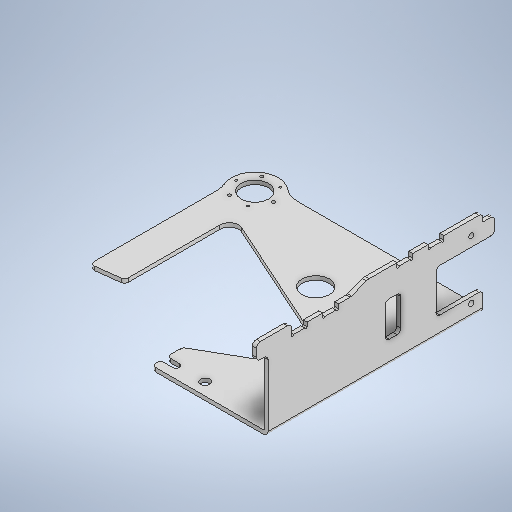
# Autodesk Inventor part: 21-30-220-A
Saved by Autodesk Inventor 2025.2 (Build 292293000, 293)
## iProperties
Created: 2024-11-14
Part Number: 21-30-220-A
Material: Generic
Document SubType Name: Sheet Metal
Designer: Zvonko.Gabric
Density: 1 g/cm^3
Appearance: Default
Sheet Metal Rule: Default
Author: Zvonko.Gabric
Autodesk Inventor part; units mm, degrees
ref_plane "YZ Plane" through (0, 0, 0) normal (1, 0, 0) x (0, 1, 0)
ref_plane "XZ Plane" through (0, 0, 0) normal (0, 1, 0) x (-1, 0, 0)
ref_plane "XY Plane" through (0, 0, 0) normal (0, 0, 1) x (1, 0, 0)
sketch "Sketch1" plane through (0, 0, 0) normal (0, 1, 0) x (-1, 0, 0)
  line L0 (0, 0) -> (140, 0)
  line L1 (145, -5) -> (145, -6)
  line L2 (140, -11) -> (129, -11)
  line L3 (129, -19.6) -> (140, -19.6)
  line L4 (145, -24.6) -> (145, -36.4)
  line L5 (142.4871, -40.7375) -> (88.5077, -71.6894)
  line L6 (257, -199.3068) -> (257, -81.9957)
  line L7 (261.3907, -77.0329) -> (291.3907, -73.3494)
  line L8 (297, -78.3121) -> (297, -235.0208)
  line L9 (0, 0) -> (-79.25, 0)
  line L10 (-84.25, 5) -> (-84.25, 10)
  line L11 (-89.25, 15) -> (-99.25, 15)
  line L12 (-104.25, 10) -> (-104.25, -24.9)
  line L13 (-99.25, -29.9) -> (-90.75, -29.9)
  arc A0 (-84.25, 5) -> (-79.25, 0) centre (-79.25, 5) ccw
  arc A1 (-84.25, 10) -> (-89.25, 15) centre (-89.25, 10) ccw
  arc A2 (-99.25, 15) -> (-104.25, 10) centre (-99.25, 10) ccw
  arc A3 (-104.25, -24.9) -> (-99.25, -29.9) centre (-99.25, -24.9) ccw
  line L14 (-90.75, -32.9) -> (-90.75, -47.1)
  arc A4 (-90.75, -50.1) -> (-90.75, -47.1) centre (-90.75, -48.6) ccw
  line L15 (-90.75, -50.1) -> (-95.85, -50.1)
  line L16 (-95.85, -69.9) -> (-90.75, -69.9)
  arc A5 (-90.75, -72.9) -> (-90.75, -69.9) centre (-90.75, -71.4) ccw
  line L17 (-90.75, -72.9) -> (-90.75, -87.1)
  arc A6 (-90.75, -90.1) -> (-90.75, -87.1) centre (-90.75, -88.6) ccw
  line L18 (-90.75, -90.1) -> (-95.85, -90.1)
  line L19 (-95.85, -90.1) -> (-95.85, -105)
  line L20 (-96.1873, -106.8055) -> (-103.5753, -125.885)
  arc A7 (-96.1873, -106.8055) -> (-95.85, -105) centre (-100.85, -105) ccw
  arc A8 (-103.5753, -125.885) -> (-104.25, -129.496) centre (-94.25, -129.496) ccw
  line L21 (-104.25, -164.9) -> (-99.15, -164.9)
  arc A9 (-99.15, -167.9) -> (-99.15, -164.9) centre (-99.15, -166.4) ccw
  line L22 (-99.15, -167.9) -> (-99.15, -182.1)
  arc A10 (-99.15, -185.1) -> (-99.15, -182.1) centre (-99.15, -183.6) ccw
  line L23 (-99.15, -185.1) -> (-104.25, -185.1)
  line L24 (-104.25, -185.1) -> (-104.25, -204.9)
  line L25 (-104.25, -204.9) -> (-99.15, -204.9)
  arc A11 (-99.15, -207.9) -> (-99.15, -204.9) centre (-99.15, -206.4) ccw
  line L26 (-99.15, -207.9) -> (-99.15, -222.1)
  arc A12 (-99.15, -225.1) -> (-99.15, -222.1) centre (-99.15, -223.6) ccw
  line L27 (-99.15, -225.1) -> (-104.25, -225.1)
  line L28 (-104.25, -225.1) -> (-104.25, -270)
  line L29 (-99.25, -275) -> (-94.25, -275)
  arc A13 (-104.25, -270) -> (-99.25, -275) centre (-99.25, -270) ccw
  line L30 (-94.25, -275) -> (-94.25, -285)
  line L31 (-89.25, -290) -> (-78.75, -290)
  line L32 (-73.75, -285) -> (-73.75, -220)
  arc A14 (-94.25, -285) -> (-89.25, -290) centre (-89.25, -285) ccw
  arc A15 (-78.75, -290) -> (-73.75, -285) centre (-78.75, -285) ccw
  line L33 (-68.75, -215) -> (-23.75, -215)
  arc A16 (-68.75, -215) -> (-73.75, -220) centre (-68.75, -220) ccw
  line L34 (-18.75, -220) -> (-18.75, -270)
  arc A17 (-18.75, -220) -> (-23.75, -215) centre (-23.75, -220) ccw
  arc A18 (145, -5) -> (140, 0) centre (140, -5) ccw
  arc A19 (140, -11) -> (145, -6) centre (140, -6) ccw
  arc A20 (129, -11) -> (129, -19.6) centre (129, -15.3) ccw
  arc A21 (145, -24.6) -> (140, -19.6) centre (140, -24.6) ccw
  arc A22 (142.4871, -40.7375) -> (145, -36.4) centre (140, -36.4) ccw
  arc A23 (88.5077, -71.6894) -> (87, -74.2919) centre (90, -74.2919) ccw
  line L35 (145, -36.4) -> (66.2414, -36.4) construction
  line L36 (87, -93.4769) -> (87, -28.4355) construction
  line L37 (88.7669, -142.0268) -> (240.0676, -210.2463)
  arc A24 (240.0676, -210.2463) -> (257, -199.3068) centre (245, -199.3068) ccw
  arc A25 (87, -139.2919) -> (88.7669, -142.0268) centre (90, -139.2919) ccw
  arc A26 (261.3907, -77.0329) -> (257, -81.9957) centre (262, -81.9957) ccw
  arc A27 (297, -78.3121) -> (291.3907, -73.3494) centre (292, -78.3121) ccw
  arc A28 (-18.75, -270) -> (-13.75, -275) centre (-13.75, -270) ccw
  circle A29 centre (272, -259) radius 17.5
  arc A30 (252.7386, -282) -> (299.5, -247.0104) centre (272, -259) ccw
  line L38 (-13.75, -275) -> (233.4773, -275)
  arc A31 (252.7386, -282) -> (233.4773, -275) centre (233.4773, -305) ccw
  arc A32 (297, -235.0208) -> (299.5, -247.0104) centre (327, -235.0208) ccw
  line L39 (-104.25, -129.496) -> (-104.25, -164.9)
  arc A33 (-90.75, -32.9) -> (-90.75, -29.9) centre (-90.75, -31.4) ccw
  circle A34 centre (126.9999, -192) radius 17.5
  circle A35 centre (92.499, -16) radius 5.9241
  circle A36 centre (-86.5, -260) radius 3.2358
  circle A37 centre (-11.5, -260) radius 3.448
  line L40 (-29.25, -170) -> (-64.25, -170)
  line L41 (-69.25, -165) -> (-69.25, -155)
  line L42 (-64.25, -150) -> (-29.25, -150)
  line L43 (-24.25, -155) -> (-24.25, -165)
  line L44 (-24.25, -170) -> (-69.25, -150) construction
  line L45 (-69.25, -170) -> (-24.25, -150) construction
  arc A38 (-24.25, -155) -> (-29.25, -150) centre (-29.25, -155) ccw
  arc A39 (-29.25, -170) -> (-24.25, -165) centre (-29.25, -165) ccw
  arc A40 (-64.25, -150) -> (-69.25, -155) centre (-64.25, -155) ccw
  arc A41 (-69.25, -165) -> (-64.25, -170) centre (-64.25, -165) ccw
  circle A42 centre (272, -259) radius 24 construction
  line L46 (296, -259) -> (237.5654, -259) construction
  circle A43 centre (296, -259) radius 1.5
  line L47 (260, -238.2154) -> (289.2173, -288.8213) construction
  circle A44 centre (260, -238.2154) radius 1.5
  line L48 (260, -279.7846) -> (289.2173, -229.1787) construction
  circle A45 centre (260, -279.7846) radius 1.5
  circle A46 centre (284, -238.2154) radius 2
  line L49 (284, -238.2154) -> (272, -259) construction
  line L50 (260, -238.2154) -> (289.2173, -288.8213) construction
  circle A47 centre (248, -259) radius 2
  line L51 (260, -279.7846) -> (289.2173, -229.1787) construction
  circle A48 centre (284, -279.7846) radius 2
  line L52 (87, -74.2919) -> (87, -139.2919)
  line L53 (-95.85, -50.1) -> (-95.85, -69.9)
  point P0 (145, 0)
  point P1 (145, -11)
  point P2 (145, -19.6)
  point P3 (145, -39.2967)
  point P4 (87, -141.2301)
  point P5 (297, -242.4169)
  point P6 (-84.25, 0)
  point P7 (-84.25, 15)
  point P8 (-104.25, 15)
  point P9 (-94.25, 15)
  point P10 (-95.85, -105.9342)
  point P11 (-104.25, -127.6275)
  point P12 (-104.25, -275)
  point P13 (-94.25, -290)
  point P14 (-73.75, -290)
  point P15 (-73.75, -215)
  point P16 (-18.75, -215)
  point P17 (-18.75, -275)
  point P18 (145, -5.5)
  point P19 (124.7, -15.3)
  point P20 (246.6228, -275)
  point P21 (-84, -290)
  point P22 (-101.7, -185.1)
  point P23 (-101.7, -164.9)
  point P24 (-95, -29.9)
  point P25 (-101.7, -225.1)
  point P26 (-101.7, -204.9)
  point P27 (-46.75, -160)
  point P28 (-24.25, -160)
  point P29 (-104.25, -147.198)
  point P30 (-18.75, -245)
  point P31 (87, -106.7919)
  dimension "d1" = 11
  dimension "d4" = 229.25
  dimension "d5" = 5
  dimension "d6" = 15
  dimension "d7" = 20
  dimension "d8" = 5
  dimension "d9" = 44.9
  dimension "d10" = 5
  dimension "d18" = 14.2
  dimension "d21" = 5
  dimension "d22" = 14.9
  dimension "d25" = 10
  dimension "d26" = 20.46
  dimension "d28" = 14.2
  dimension "d29" = 5.1
  dimension "d31" = 19.8
  dimension "d32" = 14.2
  dimension "d33" = 5.1
  dimension "d34" = 49.9
  dimension "d35" = 10
  dimension "d36" = 5
  dimension "d37" = 15
  dimension "d38" = 20.5
  dimension "d39" = 5
  dimension "d40" = 75
  dimension "d41" = 55
  dimension "d42" = 5
  dimension "d43" = 60
  dimension "d44" = 5
  dimension "d45" = 5
  dimension "d47" = 20.3
  dimension "d48" = 5
  dimension "d49" = 11.8
  dimension "d50" = 8.6
  dimension "d52" = 3
  dimension "d56" = 12
  dimension "d59" = 3
  dimension "d60" = 65
  dimension "d61" = 83
  dimension "d62" = 40
  dimension "d63" = 5
  dimension "d65" = 5
  dimension "d68" = 35
  dimension "d69" = 60
  dimension "d70" = 30
  dimension "d71" = 305
  dimension "d73" = 20.2
  dimension "d74" = 20.2
  dimension "d75" = 20.2
  dimension "d78" = 135
  dimension "d79" = 195.2
  dimension "d80" = 20.2
  dimension "d81" = 275
  dimension "d84" = 83
  dimension "d85" = 35
  dimension "d86" = 16
  dimension "d88" = 30
  dimension "d89" = 17.75
  dimension "d90" = 15
  dimension "d91" = 75
  dimension "d97" = 35
  dimension "d98" = 20
  dimension "d99" = 45
  dimension "d100" = 160
  constraints: 108 end point, 79 point on circle, 55 tangent, 49 centre point, 41 point on line, 14 midpoint, 11 perpendicular, 11 vertical, 10 horizontal, 9 equal radius, 5 coincident, 3 parallel, 1 collinear, 32 other
  measures "d1" distance of point (145, 0) point (145, -11)
  measures "d4" distance of point (-84.25, 0) point (145, 0)
  measures "d5" radius of A0
  measures "d6" distance between parallel lines of L9 L11
  measures "d7" distance of point (-84.25, 15) point (-104.25, 15)
  measures "d8" radius of A1
  measures "d9" distance from line of L13 point (-94.25, 15)
  measures "d10" radius of A3
  measures "d18" distance of L17.start L17.end
  measures "d21" radius of A7
  measures "d22" distance of L18.end L19.end
  measures "d25" radius of A8
  measures "d26" distance of L20.start L20.end
  measures "d28" distance of L22.start L22.end
  measures "d29" distance of L23.start L23.end
  measures "d31" distance of L23.end L24.end
  measures "d32" distance of L26.start L26.end
  measures "d33" distance of L27.start L27.end
  measures "d34" distance of L27.end point (-104.25, -275)
  measures "d35" distance of point (-104.25, -275) L29.end
  measures "d36" radius of A13
  measures "d37" distance of L29.end point (-94.25, -290)
  measures "d38" distance of point (-94.25, -290) point (-73.75, -290)
  measures "d39" radius of A14
  measures "d40" distance from line of point (-73.75, -215) L31
  measures "d41" distance of point (-73.75, -215) point (-18.75, -215)
  measures "d42" radius of A16
  measures "d43" distance of point (-18.75, -215) point (-18.75, -275)
  measures "d44" radius of A17
  measures "d45" radius of A18
  measures "d47" horizontal distance of point (145, -5.5) point (124.7, -15.3)
  measures "d48" radius of A21
  measures "d49" distance of L4.start L4.end
  measures "d50" distance between parallel lines of L3 L2
  measures "d52" radius of A23
  measures "d56" radius of A24
  measures "d59" radius of A25
  measures "d60" distance of L52.start L52.end
  measures "d61" angle of L6 L7
  measures "d62" distance between parallel lines of L8 L6
  measures "d63" radius of A26
  measures "d65" radius of A28
  measures "d68" diameter of A29
  measures "d69" diameter of A30
  measures "d70" radius of A31
  measures "d71" vertical distance of point (-94.25, 15) point (-84, -290)
  measures "d73" distance between parallel lines of L13 L15
  measures "d74" distance between parallel lines of L18 L16
  measures "d75" distance of point (-101.7, -185.1) point (-101.7, -164.9)
  measures "d78" distance from line of point (-101.7, -164.9) L13
  measures "d79" vertical distance of point (-95, -29.9) point (-101.7, -225.1)
  measures "d80" distance of point (-101.7, -225.1) point (-101.7, -204.9)
  measures "d81" distance between parallel lines of L38 L0
  measures "d84" distance from line of A34.centre L38
  measures "d85" diameter of A34
  measures "d86" distance from line of L0 A35.centre
  measures "d88" distance from line of A36.centre L31
  measures "d89" distance from line of L28 A36.centre
  measures "d90" distance from line of L38 A37.centre
  measures "d91" distance of A36.centre A37.centre
  measures "d97" distance between parallel lines of L39 L41
  measures "d98" distance of L45.end L44.start
  measures "d99" distance of L44.start L45.start
  measures "d100" distance from line of point (-46.75, -160) L9
extrude "Extrusion1" add sketch "Sketch1" along normal blind 5
sketch "Sketch2" plane through (0, 5, 0) normal (0, 1, 0) x (1, 0, 0)
  line L0 (-2.075, -59.618) -> (-2.075, 364.2068)
  line L1 (104.25, 129.496) -> (104.25, 164.9) projected
  point P0 (0, 0)
  dimension "d118" = 106.325
  constraints: 2 end point, 1 vertical
  measures "d118" distance between parallel lines of L1 L0
bend part "Bend Part1" radius 1 angle 90 line through (-2.075, 5, 59.618) along (0, 0, -1) centre toward (0, 1, 0) moving side (1, 0, 0) both sides no
body "Solid1"
